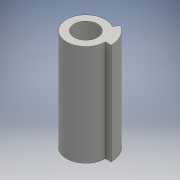
# Autodesk Inventor part: OneEdge_Drum
Saved by Autodesk Inventor 2016 (Build 200138000, 138)
## iProperties
Created: 2016-10-21
Part Number: OneEdge_Drum
Material: Generic
Document SubType Name: Modeling
Designer: Kevin
Density: 1 g/cm^3
Appearance: Default
Author: Kevin
Autodesk Inventor part; units mm, degrees
ref_plane "YZ Plane" through (0, 0, 0) normal (1, 0, 0) x (0, 1, 0)
ref_plane "XZ Plane" through (0, 0, 0) normal (0, 1, 0) x (-1, 0, 0)
ref_plane "XY Plane" through (0, 0, 0) normal (0, 0, 1) x (1, 0, 0)
sketch "Sketch1" plane through (0, 0, 0) normal (0, 0, 1) x (1, 0, 0)
  circle A0 centre (56.1598, -36.3414) radius 38.1
  circle A1 centre (56.1598, -36.3414) radius 63.5
  arc A2 (138.6898, -36.3414) -> (97.4248, 35.1317) centre (56.1598, -36.3414) ccw
  arc A3 (119.6598, -36.3414) -> (87.9098, 18.6512) centre (56.1598, -36.3414) ccw
  line L0 (97.4248, 35.1317) -> (87.9098, 18.6512)
  line L1 (138.6898, -36.3414) -> (119.6598, -36.3414)
  dimension "d19" = 76.2
  dimension "d27" = 127
  dimension "d28" = 82.53
  dimension "d29" = 82.53
  dimension "d30" = 82.53
  constraints: 6 point on circle, 4 centre point, 4 end point, 1 coincident, 1 concentric, 1 horizontal
  measures "d19" diameter of A0
  measures "d27" diameter of A1
  measures "d28" distance of A1.centre L1.start
  measures "d29" distance of A1.centre L0.start
  measures "d30" radius of A2
extrude "Extrusion4" add sketch "Sketch1" along normal blind 330.2
body "Solid4"
